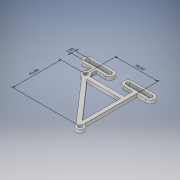
# Autodesk Inventor part: BlowerFan
Saved by Autodesk Inventor 2019 (Build 230136000, 136)
## iProperties
Created: 2018-07-02
Part Number: BlowerFan
Material: Ogólny
Document SubType Name: Modeling
Designer: Kamil
Density: 1 g/cm^3
Appearance: Domyślna
Author: Kamil
Autodesk Inventor part; units mm, degrees
ref_plane "YZ Plane" through (0, 0, 0) normal (1, 0, 0) x (0, 1, 0)
ref_plane "XZ Plane" through (0, 0, 0) normal (0, 1, 0) x (-1, 0, 0)
ref_plane "XY Plane" through (0, 0, 0) normal (0, 0, 1) x (1, 0, 0)
sketch "Szkic1" plane through (0, 0, 0) normal (0, 1, 0) x (-1, 0, 0)
  arc A0 (3.5, 0) -> (0, -3.5) centre (0, 0) ccw
  circle A1 centre (0, 0) radius 1.75
  arc A2 (34.5, -43) -> (36.25, -46.0311) centre (38, -43) ccw
  circle A3 centre (38, -43) radius 1.75
  line L0 (3.5, 0) -> (38, -39.5)
  line L1 (0, -3.5) -> (0, -43)
  line L2 (34.5, -43) -> (3.5, -43)
  line L3 (3.5, -39.5) -> (31.443, -39.5)
  line L4 (3.5, -39.5) -> (3.5, -7.5072)
  line L5 (31.443, -39.5) -> (33.443, -39.5)
  line L6 (3.5, -7.5072) -> (3.5, -6.5072)
  line L7 (3.5, -6.5072) -> (3.5, -6.0072)
  line L8 (3.5, -6.0072) -> (3.5, -5.5072)
  line L9 (3.5, -5.5072) -> (33.443, -39.5)
  line L10 (0, -43) -> (0, -50.5)
  line L11 (3.5, -43) -> (3.5, -50.5)
  line L12 (39.75, -46.0311) -> (39.75, -50.5)
  line L13 (36.25, -46.0311) -> (36.25, -50.5)
  arc A4 (39.75, -46.0311) -> (38, -39.5) centre (38, -43) ccw
  line L14 (28, -54.5) -> (48, -54.5) construction
  line L15 (28, -56.25) -> (48, -56.25)
  line L16 (48, -52.75) -> (28, -52.75)
  arc A5 (28, -52.75) -> (28, -56.25) centre (28, -54.5) ccw
  arc A6 (48, -56.25) -> (48, -52.75) centre (48, -54.5) ccw
  line L17 (38, -54.5) -> (58, -54.5) construction
  line L18 (-8.25, -54.5) -> (11.75, -54.5) construction
  line L19 (-8.25, -56.25) -> (11.75, -56.25)
  line L20 (11.75, -52.75) -> (3.5, -52.75)
  arc A7 (-8.25, -52.75) -> (-8.25, -56.25) centre (-8.25, -54.5) ccw
  arc A8 (11.75, -56.25) -> (11.75, -52.75) centre (11.75, -54.5) ccw
  line L21 (1.75, -54.5) -> (21.75, -54.5) construction
  line L22 (28, -54.5) -> (48, -54.5) construction
  line L23 (28, -58.5) -> (48, -58.5)
  line L24 (48, -50.5) -> (39.75, -50.5)
  arc A9 (28, -50.5) -> (28, -58.5) centre (28, -54.5) ccw
  arc A10 (48, -58.5) -> (48, -50.5) centre (48, -54.5) ccw
  line L25 (-8.25, -54.5) -> (11.75, -54.5) construction
  line L26 (-8.25, -58.5) -> (11.75, -58.5)
  line L27 (11.75, -50.5) -> (3.5, -50.5)
  arc A11 (-8.25, -50.5) -> (-8.25, -58.5) centre (-8.25, -54.5) ccw
  arc A12 (11.75, -58.5) -> (11.75, -50.5) centre (11.75, -54.5) ccw
  line L28 (0, -50.5) -> (-8.25, -50.5)
  line L29 (3.5, -52.75) -> (-8.25, -52.75)
  line L30 (36.25, -50.5) -> (28, -50.5)
  dimension "d0" = 7
  dimension "d1" = 3.5
  dimension "d3" = 3.5
  dimension "d4" = 2
  dimension "d5" = 1
  dimension "d6" = 0.5
  dimension "d7" = 0.5
  dimension "d10" = 10
  dimension "d12" = 3.5
  dimension "d14" = 0
  dimension "d16" = 10
  dimension "d17" = 8
  constraints: 70 end point, 23 point on circle, 22 tangent, 13 centre point, 11 parallel, 6 vertical, 5 horizontal, 4 midpoint, 3 coincident, 3 collinear, 2 perpendicular, 2 point on line
  measures "d0" diameter of A0
  measures "d1" diameter of A1
  measures "d3" diameter of A3
  measures "d4" distance of L3.end L5.end
  measures "d5" distance of L4.end L6.end
  measures "d6" distance of L6.end L7.end
  measures "d7" distance of L7.end L8.end
  measures "d10" distance of L17.start L14.end
  measures "d12" diameter of A6
  measures "d14" distance between parallel lines of L18 L21
  measures "d16" distance of L17.start L14.end
  measures "d17" diameter of A10
extrude "Wyciągnięcie proste1" add sketch "Szkic1" along normal blind 3
